Autodesk Inventor part; units mm, degrees
(part 2 of 2)
extrude "Выдавливание14" add sketch "Эскиз15" along normal blind 25.5
sketch "Эскиз16" plane through (0, 13, 0) normal (0, 1, 0) x (1, 0, 0)
  line L0 (14.893, -63.5381) -> (15, -63.3086) projected
  arc A0 (14.893, -63.5381) -> (13, -62.9053) centre (0, -104.941) ccw projected
  line L1 (13, -48.5381) -> (13, -62.9053) projected
  line L2 (15, -48.5381) -> (13, -48.5381) projected
  line L3 (15, -48.5381) -> (15, -63.3086) projected
  arc A1 (-13, -62.9053) -> (-14.893, -63.5381) centre (0, -104.941) ccw projected
  line L4 (-15, -63.3086) -> (-14.893, -63.5381) projected
  line L5 (-15, -48.5381) -> (-15, -63.3086) projected
  line L6 (-13, -48.5381) -> (-15, -48.5381) projected
  line L7 (-13, -48.5381) -> (-13, -62.9053) projected
  line L8 (8.25, -30.9214) -> (-8.25, -30.9214) projected
  point P0 (0, 0)
extrude "Выдавливание15" add sketch "Эскиз16" along normal blind 7
sketch "Эскиз17" plane through (0, 13, 0) normal (0, 1, 0) x (1, 0, 0)
  arc A0 (13, -62.9053) -> (8.25, -61.7214) centre (0, -104.941) ccw projected
  line L0 (11.5, -48.5381) -> (11.5, -66.0381) projected
  line L1 (8.25, -36.2214) -> (8.25, -61.7214) projected
  line L2 (11.5, -48.5381) -> (13, -48.5381) projected
  line L3 (11.5, -48.5381) -> (8.25, -48.5381)
  line L4 (0, -67.941) -> (0, -60.941) construction
  line L5 (-11.5, -48.5381) -> (-8.25, -48.5381)
  arc A1 (-8.25, -61.7214) -> (-13, -62.9053) centre (0, -104.941) ccw projected
  line L6 (-8.25, -36.2214) -> (-8.25, -61.7214) projected
  line L7 (-11.5, -48.5381) -> (-11.5, -66.0381) projected
  line L8 (13, -48.5381) -> (13, -62.9053) projected
  line L9 (15, -48.5381) -> (13, -48.5381) projected
  line L10 (15, -63.3086) -> (15, -48.5381) projected
  line L11 (14.893, -63.5381) -> (15, -63.3086) projected
  arc A2 (14.893, -63.5381) -> (13, -62.9053) centre (0, -104.941) ccw projected
  line L12 (-13, -62.9053) -> (-13, -48.5381) projected
  arc A3 (-13, -62.9053) -> (-14.893, -63.5381) centre (0, -104.941) ccw projected
  line L13 (-15, -63.3086) -> (-14.893, -63.5381) projected
  line L14 (-15, -48.5381) -> (-15, -63.3086) projected
  line L15 (-13, -48.5381) -> (-15, -48.5381) projected
  line L16 (-13, -48.5381) -> (-11.5, -48.5381) projected
  line L17 (-11.5, -48.5381) -> (-13, -48.5381)
  point P0 (0, 0)
  point P1 (-13, -62.9053)
  constraints: 6 end point, 3 symmetric about line, 1 collinear, 1 perpendicular, 1 point on line
extrude "Выдавливание16" add sketch "Эскиз17" along normal blind 4.5 contours A0 L0 L2 L8 | A0 L1 L3 L0 | L5 L6 A1 L7 | L7 A1 L12 L16
extrude "Выдавливание17" add sketch "Эскиз13" along normal blind 13
chamfer "Фаска1" distance 3 angle 45 1 edges at (4, 13, 40)
ref_plane "РабПлоскость4" through (14.893, 35, 48.5381) normal (0, -0.0000001, -1) x (-1, 0, 0)
sketch "Эскиз18" plane through (14.893, 35, 48.5381) normal (0, -0.0000001, -1) x (-1, 0, 0)
  line L0 (29.893, 0) -> (27.893, 0) construction
  line L1 (27.893, 0) -> (27.893, -4.5) construction
  line L2 (27.893, -4.5) -> (26.393, -6) projected
  line L3 (26.393, -6) -> (26.393, -9) projected
  line L4 (26.393, -9) -> (27.893, -9) projected
  line L5 (27.893, -9) -> (27.893, -15) construction
  line L6 (27.893, -15) -> (29.893, -15) construction
  line L7 (29.893, -15) -> (29.893, 0) construction
  line L8 (1.893, -4.5) -> (1.893, 0) construction
  line L9 (1.893, 0) -> (-0.107, 0) construction
  line L10 (-0.107, 0) -> (-0.107, -15) construction
  line L11 (-0.107, -15) -> (1.893, -15) construction
  line L12 (1.893, -15) -> (1.893, -9) construction
  line L13 (1.893, -9) -> (3.393, -9) projected
  line L14 (3.393, -9) -> (3.393, -6) projected
  line L15 (3.393, -6) -> (1.893, -4.5) projected
  line L16 (27.893, -4.5) -> (27.893, -9)
  line L17 (1.893, -4.5) -> (1.893, -9) projected
  line L18 (1.893, -9) -> (1.893, -4.5)
  line L19 (3.393, -9) -> (1.893, -9) projected
  line L20 (1.893, -9) -> (3.393, -7.5)
  line L21 (3.393, -6) -> (3.393, -9) projected
  line L22 (27.893, -9) -> (26.393, -7.5)
  line L23 (26.393, -6) -> (26.393, -9) projected
  point P0 (14.893, -35)
  point P1 (26.393, -7.5)
  point P2 (3.393, -7.5)
  constraints: 8 end point, 2 midpoint, 1 collinear, 1 vertical
extrude "Выдавливание18" cut sketch "Эскиз18" against normal blind 8 contours L16 L22 L3 L2 | L17 L15 L14 L20
extrude "Выдавливание19" cut sketch "Эскиз18" against normal blind 80 contours L4 L3 L22 | L20 L14 L13
sketch "Эскиз19" plane through (0, 17.5, 0) normal (0, 1, 0) x (1, 0, 0)
  circle A0 centre (0, -40) radius 1.9 construction
  line L0 (-5.25, -61.7214) -> (-8.25, -61.7214) construction
  line L1 (-8.25, -48.5381) -> (-8.25, -61.7214) construction
  line L2 (-8.25, -48.5381) -> (-13, -48.5381) construction
  line L3 (-13, -70.3) -> (-13, -48.5381) construction
  arc A1 (-4.5, -68.2157) -> (-13, -70.3) centre (0, -104.941) ccw construction
  line L4 (-4.5, -68.2157) -> (-4.5, -54.2214) construction
  line L5 (-4.5, -54.2214) -> (4.5, -54.2214) construction
  line L6 (4.5, -54.2214) -> (4.5, -68.2157) construction
  arc A2 (13, -70.3) -> (4.5, -68.2157) centre (0, -104.941) ccw construction
  line L7 (13, -62.9053) -> (13, -70.3) construction
  line L8 (13, -48.5381) -> (13, -62.9053) construction
  line L9 (13, -48.5381) -> (8.25, -48.5381) construction
  line L10 (8.25, -61.7214) -> (8.25, -48.5381) construction
  line L11 (8.25, -61.7214) -> (5.25, -61.7214) construction
  line L12 (5.25, -61.7214) -> (5.25, -36.2214) construction
  line L13 (5.25, -36.2214) -> (8.25, -36.2214) construction
  line L14 (8.25, -36.2214) -> (8.25, -33.9214) construction
  line L15 (8.25, -33.9214) -> (-8.25, -33.9214) construction
  line L16 (-8.25, -33.9214) -> (-8.25, -36.2214) construction
  line L17 (-8.25, -36.2214) -> (-5.25, -36.2214) construction
  line L18 (-5.25, -36.2214) -> (-5.25, -61.7214) construction
  line L19 (-4.5, -61.1717) -> (-4.5, -54.2214) construction
  line L20 (-4.5, -54.2214) -> (4.5, -54.2214)
  line L21 (4.5, -33.9214) -> (-4.5, -33.9214)
  line L22 (-8.25, -33.9214) -> (8.25, -33.9214) construction
  line L23 (4.5, -54.2214) -> (4.5, -68.2157) construction
  line L24 (-4.5, -54.2214) -> (4.5, -54.2214) construction
  line L25 (2.5, -54.2214) -> (2.5, -33.9214)
  line L26 (0, -54.2214) -> (0, -33.9214) construction
  line L27 (-2.5, -54.2214) -> (-2.5, -33.9214)
  point P0 (0, 0)
  dimension "d220" = 2
  constraints: 10 end point, 2 midpoint, 2 point on line, 2 symmetric about line, 1 collinear, 1 horizontal, 1 parallel, 1 perpendicular
  measures "d220" distance between parallel lines of L6 L25
extrude "Выдавливание20" cut sketch "Эскиз19" against normal blind 3
chamfer "Фаска2" distance 2 angle 45 2 edges at (-2.5, 17.5, 44.0714) (2.5, 17.5, 44.0714)
fillet "Сопряжение1" radius 3 1 edges at (0, 13, 60.941)
sketch "Эскиз20" plane through (14.893, 35, 48.5381) normal (0, -0.0000001, -1) x (-1, 0, 0)
  line L0 (1.893, -9) -> (1.893, -4.5) construction
  line L1 (1.893, -4.5) -> (1.893, 0) construction
  line L2 (1.893, 0) -> (-0.107, 0) construction
  line L3 (-0.107, 0) -> (-0.107, -15) construction
  line L4 (-0.107, -15) -> (1.893, -15) construction
  line L5 (1.893, -15) -> (1.893, -9) construction
  line L6 (27.893, -4.5) -> (27.893, -9) construction
  line L7 (27.893, -9) -> (27.893, -15) construction
  line L8 (27.893, -15) -> (29.893, -15) construction
  line L9 (29.893, -15) -> (29.893, 0) construction
  line L10 (29.893, 0) -> (27.893, 0) construction
  line L11 (27.893, 0) -> (27.893, -4.5) construction
  line L12 (-0.107, -22) -> (1.893, -22) construction
  line L13 (1.893, -22) -> (1.893, -17.5) construction
  line L14 (1.893, -17.5) -> (1.893, -15) construction
  line L15 (-0.107, -15) -> (1.893, -15) construction
  line L16 (-0.107, -22) -> (-0.107, -15) construction
  line L17 (1.893, -22) -> (6.643, -22) construction
  line L18 (6.643, -17.5) -> (6.643, -22) construction
  line L19 (1.893, -17.5) -> (6.643, -17.5) construction
  line L20 (1.893, -22) -> (1.893, -17.5) construction
  line L21 (27.893, -22) -> (29.893, -22) construction
  line L22 (29.893, -22) -> (29.893, -15) construction
  line L23 (27.893, -15) -> (29.893, -15) construction
  line L24 (27.893, -17.5) -> (27.893, -15) construction
  line L25 (27.893, -22) -> (27.893, -17.5) construction
  line L26 (23.143, -22) -> (27.893, -22) construction
  line L27 (27.893, -22) -> (27.893, -17.5) construction
  line L28 (23.143, -17.5) -> (27.893, -17.5) construction
  line L29 (23.143, -22) -> (23.143, -17.5) construction
  line L30 (0, -22) -> (-0.107, -22) projected
  ellipse E0 centre (14.893, 0) end of major axis (51.893, 0) minor radius 0 (-8.8896, 0) -> (1.893, 0) ccw construction
  line L31 (-0.107, -22) -> (-0.907, -22)
  line L32 (-0.907, -22) -> (-0.907, 0)
  line L33 (-0.907, 0) -> (-0.107, 0)
  line L34 (-0.107, 0) -> (-0.107, -22)
  line L35 (19.393, -22) -> (10.393, -22) construction
  line L36 (14.893, -22) -> (14.893, 0) construction
  line L37 (29.893, 0) -> (29.893, -15) construction
  line L38 (29.893, -22) -> (29.893, -15) construction
  line L39 (29.7859, -22) -> (29.893, -22)
  line L40 (29.893, -22) -> (30.693, -22)
  line L41 (30.693, -22) -> (30.693, 0)
  line L42 (30.693, 0) -> (29.893, 0)
  line L43 (29.893, 0) -> (29.893, -22)
  line L44 (-0.107, -22) -> (1.893, -22) projected
  point P0 (14.893, -35)
  point P1 (14.893, -35)
  point P2 (14.893, -35)
  dimension "d227" = 0.8
  constraints: 24 end point, 6 symmetric about line, 2 parallel, 1 coincident, 1 collinear, 1 midpoint, 1 perpendicular, 1 vertical, 2 other
  measures "d227" distance of L32.end L33.end
extrude "Выдавливание21" add sketch "Эскиз20" against normal blind 17
sketch "Эскиз21" plane through (13, 35, 62.9053) normal (-1, 0, 0) x (0, 0, 1)
  line L0 (-6.3672, -4.5) -> (-6.3672, -6) construction
  line L1 (-6.3672, -6) -> (3.1328, -6) construction
  line L2 (3.1328, -4.5) -> (3.1328, -6) projected
  line L3 (0, -4.5) -> (3.1328, -4.5) projected
  line L4 (-6.3672, -4.5) -> (0, -4.5) projected
  line L5 (-6.3672, -7.5) -> (3.1328, -7.5) construction
  line L6 (3.1328, -6) -> (3.1328, -7.5) projected
  line L7 (-6.3672, -6) -> (3.1328, -6) construction
  line L8 (-6.3672, -6) -> (-6.3672, -7.5) projected
  line L9 (3.1328, -7.5) -> (3.1328, -9) projected
  line L10 (-6.3672, -7.5) -> (3.1328, -7.5) construction
  line L11 (-6.3672, -7.5) -> (-6.3672, -9) projected
  line L12 (0, -9) -> (-6.3672, -9) construction
  line L13 (3.1328, -9) -> (0, -9) projected
  line L14 (-14.3672, -17.5) -> (0, -17.5) projected
  line L15 (0, -17.5) -> (0, -15) construction
  line L16 (-14.3672, -15) -> (0, -15) construction
  line L17 (-14.3672, -17.5) -> (-14.3672, -15) projected
  line L18 (0, -15) -> (0, -9) construction
  line L19 (0, -9) -> (-6.3672, -9) projected
  line L20 (-6.3672, -9) -> (-14.3672, -9) construction
  line L21 (-14.3672, -15) -> (-14.3672, -9) projected
  line L22 (-14.3672, -15) -> (0, -15) construction
  line L23 (-14.3672, -9) -> (-14.3672, -4.5) projected
  line L24 (-6.3672, -9) -> (-14.3672, -9) construction
  line L25 (-6.3672, -9) -> (-6.3672, -4.5) projected
  line L26 (-14.3672, -4.5) -> (-6.3672, -4.5) construction
  line L27 (0, -4.5) -> (0, 0) construction
  line L28 (-14.3672, 0) -> (0, 0) projected
  line L29 (-14.3672, -4.5) -> (-14.3672, 0) projected
  line L30 (-14.3672, -4.5) -> (-6.3672, -4.5) construction
  line L31 (-6.3672, -4.5) -> (0, -4.5) construction
  line L32 (7.3947, 0) -> (7.3947, -17.5) construction
  line L33 (0, 0) -> (7.3947, 0) projected
  line L34 (0, -4.5) -> (0, 0) construction
  line L35 (0, -4.5) -> (3.1328, -4.5) construction
  line L36 (3.1328, -4.5) -> (3.1328, -9) construction
  line L37 (3.1328, -9) -> (0, -9) construction
  line L38 (0, -15) -> (0, -9) construction
  line L39 (0, -17.5) -> (0, -15) construction
  line L40 (0, -17.5) -> (7.3947, -17.5) projected
  line L41 (7.3947, 0) -> (11.6219, 0.4264)
  line L42 (11.6219, 0.4264) -> (12.0071, -18.1627)
  line L43 (12.0071, -18.1627) -> (7.3947, -17.5)
  point P0 (-62.9053, -35)
  point P1 (-6.3672, -9)
  point P2 (-6.3672, -7.5)
  point P3 (-6.3672, -6)
  point P4 (-6.3672, -4.5)
  point P5 (3.1328, -7.5)
  constraints: 6 end point
extrude "Выдавливание22" cut sketch "Эскиз21" along normal blind 26.8 and the other way blind 0.8
sketch "Эскиз22" plane through (0, 15, 0) normal (0, -1, 0) x (1, 0, 0)
  line L0 (-26.8032, 79.1314) -> (-23.7825, 76.5969) projected
  arc A0 (-26.8032, 79.1314) -> (-31.2232, 73.7044) centre (-28.9734, 76.3855) ccw projected
  line L1 (-28.5452, 71.4571) -> (-31.2232, 73.7044) projected
  arc A1 (-28.5452, 71.4571) -> (-22.1434, 66.9191) centre (0, 104.941) ccw projected
  line L2 (-22.1434, 75.2987) -> (-22.1434, 66.9191) projected
  arc A2 (-23.7825, 76.5969) -> (-22.1434, 75.2987) centre (0, 104.941) ccw projected
  arc A3 (22.1434, 75.2987) -> (23.7825, 76.5969) centre (0, 104.941) ccw projected
  line L3 (22.1434, 66.9191) -> (22.1434, 75.2987) projected
  arc A4 (22.1434, 66.9191) -> (28.5452, 71.4571) centre (0, 104.941) ccw projected
  line L4 (31.2232, 73.7044) -> (28.5452, 71.4571) projected
  arc A5 (31.2232, 73.7044) -> (26.8032, 79.1314) centre (28.9734, 76.3855) ccw projected
  line L5 (23.7825, 76.5969) -> (26.8032, 79.1314) projected
  line L6 (-28.9734, 76.3855) -> (28.9734, 76.3855) construction
  point P0 (0, 0)
  constraints: 2 end point, 1 horizontal
extrude "Выдавливание23" add sketch "Эскиз22" along normal blind 6
ref_plane "РабПлоскость5" through (0, 35, 62.9053) normal (1, 0, 0) x (0, 0, -1)
sketch "Эскиз23" plane through (0, 35, 62.9053) normal (1, 0, 0) x (0, 0, -1)
  line L0 (-7.7055, -17.5447) -> (-7.7055, 0) construction
  line L1 (-13.6915, 0) -> (-7.7055, 0) construction
  line L2 (-13.6915, -26) -> (-13.6915, 0) construction
  line L3 (-12.3934, -26) -> (-13.6915, -26) construction
  line L4 (-12.3934, -26) -> (-12.3934, -35) construction
  line L5 (-12.3934, -35) -> (-8.1654, -35) construction
  line L6 (-8.1654, -35) -> (-8.1654, -30) construction
  line L7 (-8.1654, -30) -> (-8.1654, -30) construction
  line L8 (-8.1654, -30) -> (-8.1654, -35) construction
  line L9 (-8.1654, -35) -> (-12.3934, -35) construction
  line L10 (-12.3934, -35) -> (-12.3934, -26) construction
  line L11 (-13.6915, -26) -> (-12.3934, -26) construction
  line L12 (-13.6915, -26) -> (-13.6915, 0) construction
  line L13 (-7.7055, 0) -> (-13.6915, 0) construction
  line L14 (-7.7055, 0) -> (-7.7055, -17.5447) construction
  line L15 (-7.7055, -17.5447) -> (-7.3947, -17.5) construction
  line L16 (-5.3104, -17.5) -> (-7.3947, -17.5) construction
  line L17 (-5.3104, -22) -> (-5.3104, -17.5) construction
  line L18 (-5.3104, -22) -> (-5.3104, -22) construction
  line L19 (-5.3104, -22) -> (-5.3104, -17.5) construction
  line L20 (-7.3947, -17.5) -> (-5.3104, -17.5) construction
  line L21 (-7.3947, -17.5) -> (-7.7055, -17.5447) construction
  line L22 (-13.6915, -26) -> (-13.6915, 0) construction
  line L23 (-16.2261, 0) -> (-13.6915, 0) construction
  line L24 (-16.2261, -26) -> (-16.2261, 0) construction
  line L25 (-13.6915, -26) -> (-16.2261, -26) construction
  line L26 (-16.2261, -26) -> (-16.2261, 0) construction
  line L27 (-10.799, 0) -> (-16.2261, 0) construction
  line L28 (-10.799, -17.3211) -> (-10.799, 0) construction
  ellipse E0 centre (-13.4802, -20.8418) end of major axis (-10.1942, -17.5305) minor radius 1.6978 (-10.799, -17.3211) -> (-10.9239, -17.3262) ccw construction
  line L29 (-10.9239, -17.3262) -> (-10.9239, -17.6738) construction
  ellipse E1 centre (-13.4802, -14.1582) end of major axis (-10.1942, -17.4695) minor radius 1.6978 (-10.9239, -17.6738) -> (-10.799, -17.6789) ccw construction
  line L30 (-10.799, -26) -> (-10.799, -17.6789) construction
  line L31 (-16.2261, -26) -> (-10.799, -26) construction
  line L32 (-3.1328, -9) -> (6.3672, -9) construction
  line L33 (-3.1328, -4.5) -> (-3.1328, -9) construction
  line L34 (6.3672, -4.5) -> (-3.1328, -4.5) construction
  line L35 (6.3672, -9) -> (6.3672, -4.5) construction
  line L36 (-7.7055, -17.5447) -> (-7.7055, 0) construction
  line L37 (-7.3947, -17.5) -> (-7.7055, -17.5447) construction
  line L38 (14.3672, -17.5) -> (-7.3947, -17.5) construction
  line L39 (14.3672, -15) -> (14.3672, -17.5) construction
  line L40 (14.3672, 0) -> (14.3672, -15) construction
  line L41 (-0.2558, 0) -> (14.3672, 0) construction
  line L42 (-7.7055, 0) -> (-0.2558, 0) construction
  line L43 (-7.7055, -17.5447) -> (-16.2261, -17.5447) construction
  line L44 (-16.2261, -26) -> (-16.2261, 0) construction
  circle A0 centre (-11.9802, -21.5447) radius 2.5
  line L45 (-10.799, 0) -> (-16.9802, 0) construction
  line L46 (-16.9802, 0) -> (-16.9802, -26) construction
  line L47 (-16.9802, -26) -> (-16.9802, 0) construction
  line L48 (-16.9802, -26) -> (-16.2261, -26) construction
  point P0 (62.9053, -35)
  dimension "d237" = 5
  dimension "d238" = 4
  dimension "d239" = 5
  constraints: 6 end point, 2 point on line, 1 centre point, 1 collinear, 1 perpendicular, 2 other
  measures "d237" diameter of A0
  measures "d238" distance from line of L43 A0.centre
  measures "d239" distance from line of L47 A0.centre
extrude "Выдавливание24" cut sketch "Эскиз23" along normal mid plane 66
chamfer "Фаска3" distance 0.8 angle 45 2 edges at (-13.8, 26, 61.2881) (13.8, 26, 61.2881)
sketch "Эскиз24" plane through (-13.8, 35, 62.9053) normal (1, 0, 0) x (0, 0, -1)
  point P0 (62.9053, -35)
ref_plane "РабПлоскость6" through (0, 35, 0) normal (0, -1, 0) x (1, 0, 0)
sketch "Эскиз25" plane through (0, 35, 0) normal (0, -1, 0) x (1, 0, 0)
  line L0 (-4.5, 33.9214) -> (-4.5, 54.2214) construction
  line L1 (-4.5, 33.9214) -> (-8.25, 33.9214) construction
  line L2 (-8.25, 33.9214) -> (-8.25, 36.2214) construction
  line L3 (-8.25, 36.2214) -> (-5.25, 36.2214) construction
  line L4 (-5.25, 36.2214) -> (-5.25, 48.5381) construction
  line L5 (-5.25, 48.5381) -> (-8.25, 48.5381) construction
  line L6 (-8.25, 48.5381) -> (-13, 48.5381) construction
  line L7 (-13.8, 48.5381) -> (-13, 48.5381) construction
  line L8 (-13.8, 48.5381) -> (-13.8, 70.3) construction
  line L9 (-13.8, 70.3) -> (-13, 70.3) construction
  arc A0 (-13, 70.3) -> (-4.5, 68.2157) centre (0, 104.941) ccw construction
  line L10 (-4.5, 68.2157) -> (-4.5, 54.2214) construction
  line L11 (5.25, 48.5381) -> (5.25, 36.2214) construction
  line L12 (5.25, 36.2214) -> (8.25, 36.2214) construction
  line L13 (8.25, 36.2214) -> (8.25, 33.9214) construction
  line L14 (8.25, 33.9214) -> (4.5, 33.9214) construction
  line L15 (4.5, 54.2214) -> (4.5, 33.9214) construction
  line L16 (4.5, 54.2214) -> (4.5, 68.2157) construction
  arc A1 (4.5, 68.2157) -> (13, 70.3) centre (0, 104.941) ccw construction
  line L17 (13, 70.3) -> (13.8, 70.3) construction
  line L18 (13.8, 70.3) -> (13.8, 48.5381) construction
  line L19 (13, 48.5381) -> (13.8, 48.5381) construction
  line L20 (13, 48.5381) -> (8.25, 48.5381) construction
  line L21 (8.25, 48.5381) -> (5.25, 48.5381) construction
  line L22 (-13.8, 78.7021) -> (13.8, 78.7021)
  line L23 (13.8, 78.7021) -> (13.8, 28.4675)
  line L24 (13.8, 28.4675) -> (-13.8, 28.4675)
  line L25 (-13.8, 28.4675) -> (-13.8, 78.7021)
  point P0 (0, 0)
  constraints: 8 end point, 2 collinear, 2 parallel, 1 horizontal, 1 perpendicular
extrude "Выдавливание25" [suppressed]
sketch "Эскиз26" plane through (0, 0, 0) normal (0, -1, 0) x (1, 0, 0)
  line L0 (14.893, 71.0707) -> (14.893, 63.5381) construction
  line L1 (14.893, 63.5381) -> (16.9326, 59.1641) construction
  arc A0 (16.9326, 59.1641) -> (24.1831, 62.545) centre (20.5578, 60.8546) ccw construction
  line L2 (24.1831, 62.545) -> (22.1434, 66.9191) construction
  line L3 (22.1434, 66.9191) -> (22.1434, 75.2987) construction
  arc A1 (14.893, 71.0707) -> (22.1434, 75.2987) centre (0, 104.941) ccw construction
  circle A2 centre (20.5578, 60.8546) radius 1.9 construction
  arc A3 (-14.893, 63.5381) -> (14.893, 63.5381) centre (0, 104.941) ccw construction
  line L4 (14.893, 71.0707) -> (14.893, 63.5381) construction
  arc A4 (-14.893, 71.0707) -> (14.893, 71.0707) centre (0, 104.941) ccw construction
  line L5 (15, 48.5381) -> (13, 48.5381) construction
  line L6 (15, 63.3086) -> (15, 48.5381) construction
  line L7 (14.893, 63.5381) -> (15, 63.3086) construction
  arc A5 (4.5, 61.1717) -> (14.893, 63.5381) centre (0, 104.941) ccw construction
  arc A6 (4.5, 61.1717) -> (14.893, 63.5381) centre (0, 104.941) ccw construction
  line L8 (-15, 63.3086) -> (-14.893, 63.5381) construction
  line L9 (-15, 48.5381) -> (-15, 63.3086) construction
  line L10 (-13, 48.5381) -> (-15, 48.5381) construction
  arc A7 (-14.893, 71.0707) -> (14.893, 71.0707) centre (0, 104.941) ccw construction
  line L11 (-14.893, 63.5381) -> (-14.893, 71.0707) construction
  arc A8 (-14.893, 63.5381) -> (14.893, 63.5381) centre (0, 104.941) ccw construction
  circle A9 centre (0, 40) radius 4 construction
  circle A10 centre (0, 40) radius 1.9 construction
  line L12 (14.893, 71.0707) -> (14.893, 63.5381) projected
  line L13 (4.5, 54.2214) -> (4.5, 61.1717) projected
  line L14 (-4.5, 54.2214) -> (4.5, 54.2214) projected
  line L15 (-4.5, 61.1717) -> (-4.5, 54.2214) projected
  arc A11 (-14.893, 63.5381) -> (-4.5, 61.1717) centre (0, 104.941) ccw projected
  line L16 (-8.25, 48.5381) -> (-13, 48.5381) projected
  line L17 (-8.25, 30.9214) -> (-8.25, 48.5381) projected
  line L18 (8.25, 30.9214) -> (-8.25, 30.9214) projected
  line L19 (8.25, 48.5381) -> (8.25, 30.9214) projected
  line L20 (13, 48.5381) -> (8.25, 48.5381) projected
  line L21 (15, 48.5381) -> (13, 48.5381) projected
  line L22 (15, 63.3086) -> (15, 48.5381) projected
  line L23 (14.893, 63.5381) -> (15, 63.3086) projected
  line L24 (4.5, 54.2214) -> (4.5, 61.1717) projected
  line L25 (-4.5, 54.2214) -> (4.5, 54.2214) projected
  line L26 (-4.5, 61.1717) -> (-4.5, 54.2214) projected
  arc A12 (-14.893, 63.5381) -> (-4.5, 61.1717) centre (0, 104.941) ccw projected
  line L27 (-15, 63.3086) -> (-14.893, 63.5381) projected
  line L28 (-15, 48.5381) -> (-15, 63.3086) projected
  line L29 (-13, 48.5381) -> (-15, 48.5381) projected
  line L30 (-8.25, 48.5381) -> (-13, 48.5381) projected
  line L31 (-8.25, 30.9214) -> (-8.25, 48.5381) projected
  line L32 (8.25, 30.9214) -> (-8.25, 30.9214) projected
  line L33 (8.25, 48.5381) -> (8.25, 30.9214) projected
  line L34 (13, 48.5381) -> (8.25, 48.5381) projected
  line L35 (-14.893, 63.5381) -> (-14.893, 71.0707) projected
  point P0 (0, 0)
ref_plane "РабПлоскость7" through (0, 11, 0) normal (0, -1, 0) x (1, 0, 0)
sketch "Эскиз27" plane through (0, 11, 0) normal (0, -1, 0) x (1, 0, 0)
  arc A0 (4.5, 61.1717) -> (14.893, 63.5381) centre (0, 104.941) ccw projected
  line L0 (4.5, 54.2214) -> (4.5, 61.1717) projected
  line L1 (-4.5, 54.2214) -> (4.5, 54.2214) projected
  line L2 (-4.5, 61.1717) -> (-4.5, 54.2214) projected
  arc A1 (-14.893, 63.5381) -> (-4.5, 61.1717) centre (0, 104.941) ccw projected
  line L3 (-15, 63.3086) -> (-14.893, 63.5381) projected
  line L4 (-15, 48.5381) -> (-15, 63.3086) projected
  line L5 (-13, 48.5381) -> (-15, 48.5381) projected
  line L6 (-8.25, 48.5381) -> (-13, 48.5381) projected
  line L7 (-8.25, 30.9214) -> (-8.25, 48.5381) projected
  line L8 (8.25, 30.9214) -> (-8.25, 30.9214) projected
  line L9 (8.25, 48.5381) -> (8.25, 30.9214) projected
  line L10 (13, 48.5381) -> (8.25, 48.5381) projected
  line L11 (15, 48.5381) -> (13, 48.5381) projected
  line L12 (15, 63.3086) -> (15, 48.5381) projected
  line L13 (14.893, 63.5381) -> (15, 63.3086) projected
  circle A2 centre (0, 40) radius 7 projected
  circle A3 centre (0, 40) radius 1.9 projected
  circle A4 centre (0, 40) radius 4 projected
  circle A5 centre (0, 40) radius 1.9 projected
  line L14 (-15.8, 61.593) -> (-15, 63.3086) projected
  line L15 (-15.8, 48.5381) -> (-15.8, 61.593) projected
  line L16 (-15, 48.5381) -> (-15.8, 48.5381) projected
  line L17 (-15, 48.5381) -> (-15, 63.3086) projected
  line L18 (15, 63.3086) -> (15.8, 61.593) projected
  line L19 (15, 63.3086) -> (15, 48.5381) projected
  line L20 (15.8, 48.5381) -> (15, 48.5381) projected
  line L21 (15.8, 48.5381) -> (15.8, 61.593) projected
  line L22 (13.8, 48.5381) -> (13.8, 63.1611) projected
  line L23 (5.25, 48.5381) -> (5.25, 36.2214) projected
  line L24 (5.25, 36.2214) -> (8.25, 36.2214) projected
  line L25 (8.25, 36.2214) -> (8.25, 33.9214) projected
  line L26 (8.25, 33.9214) -> (4.5, 33.9214) projected
  line L27 (4.5, 54.2214) -> (4.5, 33.9214) projected
  line L28 (4.5, 54.2214) -> (4.5, 68.2157) projected
  arc A6 (4.5, 68.2157) -> (13, 70.3) centre (0, 104.941) ccw projected
  line L29 (13, 70.3) -> (13.8, 70.3) projected
  line L30 (13.8, 70.3) -> (13.8, 48.5381) projected
  line L31 (13, 48.5381) -> (13.8, 48.5381) projected
  line L32 (13, 48.5381) -> (8.25, 48.5381) projected
  line L33 (8.25, 48.5381) -> (5.25, 48.5381) projected
  line L34 (-4.5, 33.9214) -> (-4.5, 54.2214) projected
  line L35 (-4.5, 33.9214) -> (-8.25, 33.9214) projected
  line L36 (-8.25, 33.9214) -> (-8.25, 36.2214) projected
  line L37 (-8.25, 36.2214) -> (-5.25, 36.2214) projected
  line L38 (-5.25, 36.2214) -> (-5.25, 48.5381) projected
  line L39 (-5.25, 48.5381) -> (-8.25, 48.5381) projected
  line L40 (-8.25, 48.5381) -> (-13, 48.5381) projected
  line L41 (-13.8, 48.5381) -> (-13, 48.5381) projected
  line L42 (-13.8, 48.5381) -> (-13.8, 70.3) projected
  line L43 (-13.8, 70.3) -> (-13, 70.3) projected
  arc A7 (-13, 70.3) -> (-4.5, 68.2157) centre (0, 104.941) ccw projected
  line L44 (-4.5, 68.2157) -> (-4.5, 54.2214) projected
  point P0 (0, 0)
  point P1 (-13.8, 48.5381)
  point P2 (-13.8, 63.1611)
extrude "Выдавливание26" add sketch "Эскиз27" along normal blind 6 contours A0 L22 L11 L10 L33 L23 A2 L27 L0 | A0 L13 L12 L11 L22 | L27 A2 L34 L1 | L34 A2 L38 L39 L6 L5 L42 A1 L2 | L27 A2 L34 | A2 L23 L24 L27 | L18 L21 L20 L12 | L34 A2 L37 L38 | L23 L33 L9 L24 A2 | A2 L24 L23 | L27 L26 L9 L8 L7 L35 L34 A2 | A2 L24 L9 L26 L27 | L42 L5 L4 L3 A1 | L38 L37 A2 | A2 L37 L7 L39 L38 | L34 L35 L7 L37 A2 | L4 L16 L15 L14 | A4
sketch "Эскиз28" plane through (0, 35, 0) normal (0, -1, 0) x (1, 0, 0)
  line L0 (-4.5, 33.9214) -> (-4.5, 54.2214) construction
  line L1 (-4.5, 33.9214) -> (-8.25, 33.9214) construction
  line L2 (-8.25, 33.9214) -> (-8.25, 36.2214) construction
  line L3 (-8.25, 36.2214) -> (-5.25, 36.2214) construction
  line L4 (-5.25, 36.2214) -> (-5.25, 48.5381) construction
  line L5 (-5.25, 48.5381) -> (-8.25, 48.5381) construction
  line L6 (-8.25, 48.5381) -> (-13, 48.5381) construction
  line L7 (-13.8, 48.5381) -> (-13, 48.5381) construction
  line L8 (-13.8, 48.5381) -> (-13.8, 70.3) construction
  line L9 (-13.8, 70.3) -> (-13, 70.3) construction
  arc A0 (-13, 70.3) -> (-4.5, 68.2157) centre (0, 104.941) ccw construction
  line L10 (-4.5, 68.2157) -> (-4.5, 54.2214) construction
  line L11 (-8.25, 30.9214) -> (-8.25, 33.9214) construction
  line L12 (-8.25, 33.9214) -> (8.25, 33.9214) construction
  line L13 (8.25, 33.9214) -> (8.25, 30.9214) construction
  line L14 (8.25, 30.9214) -> (-8.25, 30.9214) construction
  line L15 (5.25, 48.5381) -> (5.25, 36.2214) construction
  line L16 (5.25, 36.2214) -> (8.25, 36.2214) construction
  line L17 (8.25, 36.2214) -> (8.25, 33.9214) construction
  line L18 (8.25, 33.9214) -> (4.5, 33.9214) construction
  line L19 (4.5, 54.2214) -> (4.5, 33.9214) construction
  line L20 (4.5, 54.2214) -> (4.5, 68.2157) construction
  arc A1 (4.5, 68.2157) -> (13, 70.3) centre (0, 104.941) ccw construction
  line L21 (13, 70.3) -> (13.8, 70.3) construction
  line L22 (13.8, 70.3) -> (13.8, 48.5381) construction
  line L23 (13, 48.5381) -> (13.8, 48.5381) construction
  line L24 (13, 48.5381) -> (8.25, 48.5381) construction
  line L25 (8.25, 48.5381) -> (5.25, 48.5381) construction
  line L26 (-13.8, 84.9747) -> (13.8, 84.9747)
  line L27 (13.8, 84.9747) -> (13.8, 27.4601)
  line L28 (13.8, 27.4601) -> (-13.8, 27.4601)
  line L29 (-13.8, 27.4601) -> (-13.8, 84.9747)
  line L30 (13.8, 63.1611) -> (13.8, 70.6109) projected
  point P0 (0, 0)
  constraints: 8 end point, 2 collinear, 2 parallel, 1 horizontal, 1 perpendicular
extrude "Выдавливание27" cut sketch "Эскиз28" along normal blind 27
extrude "Выдавливание28" add sketch "Эскиз27" against normal blind 3 contours A0 L13 L12 L11 L22 | L18 L21 L20 L12 | L42 L5 L4 L3 A1 | L4 L16 L15 L14
chamfer "Фаска4" distance 1 angle 45 1 edges at (4, 5, 40)
ref_plane "РабПлоскость8" through (30.8, 19.82, 61.593) normal (1, 0, 0) x (0, 0, -1)
sketch "Эскиз29" plane through (30.8, 19.82, 61.593) normal (1, 0, 0) x (0, 0, -1)
  arc A0 (-12.1114, -8.5681) -> (-12.1114, -4.1613) centre (-13.2925, -6.3647) ccw construction
  circle A1 centre (-13.2925, -6.3647) radius 3.5
  point P0 (61.593, -19.82)
  dimension "d259" = 7
  constraints: 1 centre point, 1 coincident, 1 vertical alignment
  measures "d259" diameter of A1
extrude "Выдавливание29" cut sketch "Эскиз29" along normal blind 3
ref_plane "РабПлоскость9" through (24.8, 35, 62.9053) normal (-1, 0, 0) x (0, 0, 1)
sketch "Эскиз30" plane through (24.8, 35, 62.9053) normal (-1, 0, 0) x (0, 0, 1)
  line L0 (10.4439, -23.5169) -> (10.4439, -24.6895) construction
  arc A0 (10.4439, -23.5169) -> (10.4439, -19.5724) centre (11.9802, -21.5447) ccw projected
  line L1 (10.4439, -18.3998) -> (10.4439, -19.5724) construction
  arc A1 (10.4439, -24.6895) -> (10.4439, -18.3998) centre (11.9802, -21.5447) ccw construction
  line L2 (10.799, -18.25) -> (10.799, 0) construction
  line L3 (16.2261, 0) -> (10.799, 0) construction
  line L4 (16.2261, -26) -> (16.2261, 0) construction
  line L5 (10.799, -26) -> (16.2261, -26) construction
  line L6 (10.799, -26) -> (10.799, -24.8394) construction
  line L7 (13.4802, -19.5447) -> (13.4802, -23.5447)
  point P0 (-62.9053, -35)
  dimension "d263" = 1.5
  constraints: 2 end point, 2 point on circle, 1 vertical, 1 vertical alignment
  measures "d263" distance from line of A0.centre L7
extrude "Выдавливание30" add sketch "Эскиз30" against normal blind 2
chamfer "Фаска5" distance 0.7 angle 45 1 edges at (26.8, 13.4553, 76.3855)
fillet "Сопряжение2" radius 8 2 edges at (-8.25, 6.5, 30.9214) (8.25, 6.5, 30.9214)
fillet "Сопряжение3" radius 5 2 edges at (8.25, 6.5, 48.5381) (-8.25, 6.5, 48.5381)
ref_plane "РабПлоскость10" through (30.8, 15.4276, 73.3492) normal (0, 0, 1) x (1, 0, 0)
sketch "Эскиз31" plane through (30.8, 15.4276, 73.3492) normal (0, 0, 1) x (1, 0, 0)
  line L0 (-53.2578, 14.5724) -> (-49.4578, 14.5724) construction
  line L1 (-46.6, 19.5724) -> (-46.6, 4.3924) construction
  line L2 (-17, 19.5724) -> (-17, -7.4276) construction
  line L3 (-17, -7.4276) -> (-44.6, -7.4276) construction
  line L4 (-44.6, -7.4276) -> (-44.6, 19.5724) construction
  line L5 (-54.5825, 19.5724) -> (-44.6, 19.5724) construction
  line L6 (-54.5825, -0.1499) -> (-54.5825, 19.5724) construction
  line L7 (-54.5825, -6.4276) -> (-54.5825, -3.7947) construction
  line L8 (-52.9434, -6.4276) -> (-54.5825, -6.4276) construction
  line L9 (-52.9434, -6.4276) -> (-52.9434, -15.4276) construction
  line L10 (-52.9434, -15.4276) -> (-45.693, -15.4276) construction
  line L11 (-45.693, -15.4276) -> (-45.693, -10.4276) construction
  line L12 (-15.907, -10.4276) -> (-45.693, -10.4276) construction
  line L13 (-15.907, -10.4276) -> (-15.907, -15.4276) construction
  line L14 (-15.907, -15.4276) -> (-8.6566, -15.4276) construction
  line L15 (-8.6566, -15.4276) -> (-8.6566, -6.4276) construction
  line L16 (-7.0175, -6.4276) -> (-8.6566, -6.4276) construction
  line L17 (-7.0175, -6.4276) -> (-7.0175, -3.7947) construction
  line L18 (-7.0175, -0.1499) -> (-7.0175, 19.5724) construction
  line L19 (-17, 19.5724) -> (-7.0175, 19.5724) construction
  line L20 (-30.8, -15.4276) -> (-30.8, 19.5724) construction
  line L21 (-15, 19.5724) -> (-15, -2.4276) construction
  line L22 (-21.4323, 12.5724) -> (-11, 12.5724)
  line L23 (-11, 12.5724) -> (-11, 2.5724)
  line L24 (-11, 2.5724) -> (-21.4323, 2.5724)
  line L25 (-21.4323, 2.5724) -> (-21.4323, 12.5724)
  line L26 (-40.1677, 12.5724) -> (-50.6, 12.5724)
  line L27 (-50.6, 12.5724) -> (-50.6, 2.5724)
  line L28 (-50.6, 2.5724) -> (-40.1677, 2.5724)
  line L29 (-40.1677, 2.5724) -> (-40.1677, 12.5724)
  dimension "d273" = 7
  dimension "d274" = 10
  dimension "d275" = 6
  constraints: 18 end point, 4 symmetric about line, 2 parallel, 2 vertical alignment, 1 horizontal, 1 perpendicular, 1 vertical
  measures "d273" distance between parallel lines of L19 L22
  measures "d274" distance between parallel lines of L22 L24
  measures "d275" distance between parallel lines of L2 L23
extrude "Выдавливание31" cut sketch "Эскиз31" against normal blind 18
sketch "Эскиз32" plane through (0, 0, 0) normal (0, -1, 0) x (1, 0, 0)
  line L0 (22.1434, 66.9191) -> (22.1434, 75.2987) construction
  arc A0 (22.1434, 66.9191) -> (28.5452, 71.4571) centre (0, 104.941) ccw construction
  line L1 (28.5452, 71.4571) -> (31.2232, 73.7044) construction
  arc A1 (31.2232, 73.7044) -> (26.8032, 79.1314) centre (28.9734, 76.3855) ccw construction
  line L2 (26.8032, 79.1314) -> (23.7825, 76.5969) construction
  arc A2 (22.1434, 75.2987) -> (23.7825, 76.5969) centre (0, 104.941) ccw construction
  line L3 (-29.6515, 72.3855) -> (-17.5823, 72.3855) construction
  arc A3 (-26.8032, 79.1314) -> (-31.2232, 73.7044) centre (-28.9734, 76.3855) ccw construction
  line L4 (-31.2232, 73.7044) -> (-28.5452, 71.4571) construction
  arc A4 (-28.5452, 71.4571) -> (-22.1434, 66.9191) centre (0, 104.941) ccw construction
  line L5 (-22.1434, 75.2987) -> (-22.1434, 66.9191) construction
  arc A5 (-23.7825, 76.5969) -> (-22.1434, 75.2987) centre (0, 104.941) ccw construction
  line L6 (-23.7825, 76.5969) -> (-26.8032, 79.1314) construction
  circle A6 centre (-20.5578, 60.8546) radius 1.9 construction
  line L7 (-14.893, 63.5381) -> (-14.893, 71.0707) construction
  arc A7 (-22.1434, 75.2987) -> (-14.893, 71.0707) centre (0, 104.941) ccw construction
  line L8 (-22.1434, 75.2987) -> (-22.1434, 66.9191) construction
  line L9 (-22.1434, 66.9191) -> (-24.1831, 62.545) construction
  arc A8 (-24.1831, 62.545) -> (-16.9326, 59.1641) centre (-20.5578, 60.8546) ccw construction
  line L10 (-16.9326, 59.1641) -> (-14.893, 63.5381) construction
  arc A9 (15.8, 63.8757) -> (22.1434, 66.9191) centre (0, 104.941) ccw construction
  line L11 (14.893, 71.0707) -> (14.893, 63.5381) construction
  line L12 (14.893, 63.5381) -> (16.9326, 59.1641) construction
  arc A10 (16.9326, 59.1641) -> (24.1831, 62.545) centre (20.5578, 60.8546) ccw construction
  line L13 (24.1831, 62.545) -> (22.1434, 66.9191) construction
  line L14 (22.1434, 66.9191) -> (22.1434, 75.2987) construction
  arc A11 (14.893, 71.0707) -> (22.1434, 75.2987) centre (0, 104.941) ccw construction
  circle A12 centre (20.5578, 60.8546) radius 1.9 construction
  line L15 (28.9734, 76.3855) -> (0, 56.6418) construction
  circle A13 centre (0, 40) radius 4 construction
  circle A14 centre (0, 40) radius 1.9 construction
  line L16 (14.893, 71.0707) -> (14.893, 63.5381) construction
  arc A15 (-14.893, 71.0707) -> (14.893, 71.0707) centre (0, 104.941) ccw construction
  line L17 (-14.893, 63.5381) -> (-14.893, 71.0707) construction
  arc A16 (-4.5, 61.1717) -> (4.5, 61.1717) centre (0, 104.941) ccw construction
  line L18 (0, 40) -> (0, 67.941) construction
  arc A17 (-13.8, 70.6109) -> (13.8, 70.6109) centre (0, 104.941) ccw construction
  line L19 (-28.9734, 76.3855) -> (0, 56.6418) construction
  line L20 (34.2533, 72.083) -> (25.8539, 84.409)
  line L21 (-34.2533, 72.083) -> (-25.8539, 84.409)
  line L22 (34.2533, 72.083) -> (35.2275, 83.2669)
  line L23 (35.2275, 83.2669) -> (25.8539, 84.409)
  line L24 (-25.8539, 84.409) -> (-35.9095, 83.2669)
  line L25 (-35.9095, 83.2669) -> (-34.2533, 72.083)
  arc A18 (0.25, 30.9214) -> (8.25, 38.9214) centre (0.25, 38.9214) ccw projected
  line L26 (8.25, 38.9214) -> (8.25, 43.5381) projected
  arc A19 (13.25, 48.5381) -> (8.25, 43.5381) centre (13.25, 43.5381) ccw projected
  line L27 (13.25, 48.5381) -> (15.8, 48.5381) projected
  line L28 (15.8, 48.5381) -> (15.8, 61.593) projected
  line L29 (14.893, 63.5381) -> (15.8, 61.593) projected
  line L30 (-15.8, 61.593) -> (-14.893, 63.5381) projected
  line L31 (-15.8, 61.593) -> (-15.8, 48.5381) projected
  line L32 (-15.8, 48.5381) -> (-13.25, 48.5381) projected
  arc A20 (-8.25, 43.5381) -> (-13.25, 48.5381) centre (-13.25, 43.5381) ccw projected
  line L33 (-8.25, 43.5381) -> (-8.25, 38.9214) projected
  arc A21 (-8.25, 38.9214) -> (-0.25, 30.9214) centre (-0.25, 38.9214) ccw projected
  line L34 (-0.25, 30.9214) -> (0.25, 30.9214) projected
  line L35 (4.5, 61.1717) -> (4.5, 54.2214) projected
  line L36 (4.5, 54.2214) -> (-4.5, 54.2214) projected
  line L37 (-4.5, 54.2214) -> (-4.5, 61.1717) projected
  point P0 (0, 0)
  constraints: 18 end point, 3 symmetric about line, 2 point on circle, 1 perpendicular, 3 other
extrude "Выдавливание32" cut sketch "Эскиз32" against normal up to surface (35 mm away)
